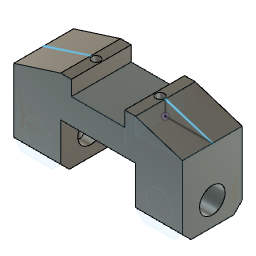
Antena (Autodesk Fusion 360 design; units mm, degrees)
Autodesk Fusion 360 part; units mm, degrees
sketch "Sketch1" plane through (0, 0, 0) normal (0, 0, 1) x (1, 0, 0)
  line L0 (-125, 140) -> (125, 140)
  line L1 (125, 140) -> (125, -140)
  line L2 (125, -140) -> (-125, -140)
  line L3 (-125, -140) -> (-125, 140)
  line L4 (-125, 140) -> (-175, 140)
  line L5 (-175, 140) -> (-175, -140)
  line L6 (-175, -140) -> (-125, -140)
  line L7 (-125, -140) -> (-125, 140)
  line L8 (-175, 140) -> (-425, 140)
  line L9 (-425, 140) -> (-425, -140)
  line L10 (-425, -140) -> (-175, -140)
  line L11 (-175, -140) -> (-175, 140)
  line L12 (125, 140) -> (175, 140)
  line L13 (175, 140) -> (175, -140)
  line L14 (175, -140) -> (125, -140)
  line L15 (125, -140) -> (125, 140)
  line L16 (175, 140) -> (425, 140)
  line L17 (425, 140) -> (425, -140)
  line L18 (425, -140) -> (175, -140)
  line L19 (175, -140) -> (175, 140)
  point P0 (-125, 140)
  dimension "d1" = 250
  dimension "d2" = 280
  dimension "d3" = 50
  dimension "d4" = 280
  dimension "d5" = 250
  dimension "d6" = 280
  dimension "d7" = 50
  dimension "d8" = 280
  dimension "d9" = 250
  dimension "d10" = 280
  constraint horizontal L0
  constraint vertical L1
  constraint horizontal L2
  constraint vertical L3
  constraint coincident P0 L0.start
  constraint horizontal L4
  constraint vertical L5
  constraint horizontal L6
  constraint vertical L7
  constraint horizontal L8
  constraint vertical L9
  constraint horizontal L10
  constraint vertical L11
  constraint horizontal L12
  constraint vertical L13
  constraint horizontal L14
  constraint vertical L15
  constraint horizontal L16
  constraint vertical L17
  constraint horizontal L18
  constraint vertical L19
  measures "d1" distance of P0 L0.end
  measures "d2" distance of P0 L2.end
  measures "d3" distance of P0 L4.end
  measures "d4" distance of P0 L2.end
  measures "d5" distance of L4.end L8.end
  measures "d6" distance of L4.end L5.end
  measures "d7" distance of L0.end L12.end
  measures "d8" distance of L0.end L1.end
  measures "d9" distance of L12.end L16.end
  measures "d10" distance of L12.end L13.end
extrude "Extrude1" add sketch "Sketch1" against normal blind 60 contours L0 L1 L2 L3 L7 L15 makes body 1
sketch "Sketch2" plane through (125, 0, 0) normal (1, 0, 0) x (0, 1, 0)
  line L0 (140, 0) -> (-140, 0)
  line L1 (-140, 0) -> (-140, -60)
  line L2 (-140, -60) -> (140, -60)
  line L3 (140, -60) -> (140, 0)
sketch "Sketch3" plane through (0, 0, 0) normal (0, 0, 1) x (1, 0, 0)
  line L0 (-125, 140) -> (-175, 140)
  line L1 (-175, 140) -> (-175, -140)
  line L2 (-175, -140) -> (-125, -140)
  line L3 (-125, -140) -> (-125, 140)
  line L4 (125, 140) -> (175, 140)
  line L5 (175, 140) -> (175, -140)
  line L6 (175, -140) -> (125, -140)
  line L7 (125, -140) -> (125, 140)
  dimension "d13" = 50
  dimension "d14" = 280
  dimension "d15" = 50
  dimension "d16" = 280
  constraint horizontal L0
  constraint vertical L1
  constraint horizontal L2
  constraint vertical L3
  constraint horizontal L4
  constraint vertical L5
  constraint horizontal L6
  constraint vertical L7
  measures "d13" distance of L0.start L0.end
  measures "d14" distance of L0.start L2.end
  measures "d15" distance of L4.start L4.end
  measures "d16" distance of L4.start L6.end
extrude "Extrude2" add sketch "Sketch3" along normal blind 70 separate body makes body 2 at (-125, -46.6667, 23.3333) makes body 3 at (175, 46.6667, 23.3333)
extrude "Extrude3" add 1 faces at (141.6667, 46.6667, 0) along direction (0, 0, -1) blind 60 on bodies 3 bodies 3 2 1
extrude "Extrude4" add 1 faces at (-158.3333, 46.6667, 0) along direction (0, 0, -1) blind 60 on bodies 2 bodies 2 3
sketch "Sketch4" plane through (0, 0, 0) normal (0, 0, 1) x (1, 0, 0)
  line L0 (-175, 140) -> (-395, 140)
  line L1 (-395, 140) -> (-395, -140)
  line L2 (-395, -140) -> (-175, -140)
  line L3 (-175, -140) -> (-175, 140)
  line L4 (175, 140) -> (395, 140)
  line L5 (395, 140) -> (395, -140)
  line L6 (395, -140) -> (175, -140)
  line L7 (175, -140) -> (175, 140)
  dimension "d23" = 220
  dimension "d24" = 280
  dimension "d25" = 220
  dimension "d26" = 280
  constraint horizontal L0
  constraint vertical L1
  constraint horizontal L2
  constraint vertical L3
  constraint horizontal L4
  constraint vertical L5
  constraint horizontal L6
  constraint vertical L7
  measures "d23" distance of L0.start L0.end
  measures "d24" distance of L0.start L2.end
  measures "d25" distance of L4.start L4.end
  measures "d26" distance of L4.start L6.end
extrude "Extrude5" add sketch "Sketch4" against normal blind 60 bodies 2
sketch "Sketch5" plane through (0, 0, 0) normal (0, 1, 0) x (1, 0, 0)
  line L0 (-175, -70) -> (-395, 0)
  line L1 (395, 0) -> (175, -70)
  line L2 (175, -70) -> (395, 0)
  line L3 (-175, -70) -> (-395, 0)
  constraint parallel L1 L2
sketch "Sketch6" plane through (0, 0, 0) normal (0, 0, 1) x (-1, 0, 0)
  line L0 (-175, 140) -> (-395, 140)
  line L1 (-395, 140) -> (-395, -140)
  line L2 (-395, -140) -> (-175, -140)
  line L3 (-175, -140) -> (-175, 140)
  line L4 (-175, 0) -> (-395, 0)
  constraint midpoint L3 L4.start
  constraint midpoint L1 L4.end
sketch "Sketch7" plane through (175, 0, 0) normal (1, 0, 0) x (0, 1, 0)
  line L0 (-140, 0) -> (140, 0)
  line L1 (140, 0) -> (140, 70)
  line L2 (140, 70) -> (-140, 70)
  line L3 (-140, 70) -> (-140, 0)
  line L4 (0, 70) -> (0, 0)
  constraint midpoint L2 L4.start
  constraint coincident L4.end origin
sketch "Sketch8" plane through (0, 0, 0) normal (0, 1, 0) x (1, 0, 0)
sketch "Sketch9" plane through (0, 0, 0) normal (0, 0, 1) x (-1, 0, 0)
sketch "Sketch10" plane through (0, -140, 0) normal (0, -1, 0) x (1, 0, 0)
  line L0 (-125, 0) -> (-125, 70)
  line L1 (-125, 70) -> (-175, 70)
  line L2 (-175, 70) -> (-175, 0)
  line L3 (-175, 0) -> (-395, 0)
  line L4 (-395, 0) -> (-395, -60)
  line L5 (-395, -60) -> (395, -60)
  line L6 (395, -60) -> (395, 0)
  line L7 (395, 0) -> (175, 0)
  line L8 (175, 0) -> (175, 70)
  line L9 (175, 70) -> (125, 70)
  line L10 (125, 70) -> (125, 0)
  line L11 (125, 0) -> (-125, 0)
  line L12 (175, 70) -> (395, 0)
  constraint coincident L8.end L9.start
  constraint coincident L6.end L7.start
extrude "Extrude6" add sketch "Sketch10" against normal blind 280 contours L7 L8 L12 bodies 2
sketch "Sketch11" plane through (0, -140, 0) normal (0, -1, 0) x (1, 0, 0)
  line L0 (-125, 0) -> (-125, 70)
  line L1 (-125, 70) -> (-175, 70)
  line L2 (-175, 70) -> (-175, 0)
  line L3 (-175, 0) -> (-395, 0)
  line L4 (-395, 0) -> (-395, -60)
  line L5 (-395, -60) -> (395, -60)
  line L6 (395, -60) -> (395, 0)
  line L7 (395, 0) -> (175, 70)
  line L8 (175, 70) -> (125, 70)
  line L9 (125, 70) -> (125, 0)
  line L10 (125, 0) -> (-125, 0)
  line L11 (-175, 70) -> (-395, 0)
  constraint coincident L1.end L2.start
  constraint coincident L3.end L4.start
extrude "Extrude7" add sketch "Sketch11" against normal blind 280 contours L2 L3 L11 bodies 2
sketch "Sketch12" plane through (0, 0, 0) normal (0, 0, 1) x (-1, 0, 0)
  line L0 (125, 140) -> (-125, 140)
  line L1 (-125, 140) -> (-125, -140)
  line L2 (-125, -140) -> (125, -140)
  line L3 (125, -140) -> (125, 140)
sketch "Sketch13" plane through (0, 0, -60) normal (0, 0, -1) x (1, 0, 0)
  line L0 (395, 140) -> (-395, 140)
  line L1 (-395, 140) -> (-395, -140)
  line L2 (-395, -140) -> (395, -140)
  line L3 (395, -140) -> (395, 140)
  line L4 (-395, 140) -> (-175, 140)
  line L5 (-175, 140) -> (-175, -140)
  line L6 (-175, -140) -> (-395, -140)
  line L7 (-395, -140) -> (-395, 140)
  line L8 (395, 140) -> (175, 140)
  line L9 (175, 140) -> (175, -140)
  line L10 (175, -140) -> (395, -140)
  line L11 (395, -140) -> (395, 140)
  dimension "d33" = 220
  dimension "d34" = 280
  dimension "d35" = 220
  dimension "d36" = 280
  constraint horizontal L4
  constraint vertical L5
  constraint horizontal L6
  constraint vertical L7
  constraint coincident L0.end L1.start
  constraint horizontal L8
  constraint vertical L9
  constraint horizontal L10
  constraint vertical L11
  constraint coincident L0.start L3.end
  measures "d33" distance of L0.end L4.end
  measures "d34" distance of L0.end L1.end
  measures "d35" distance of L0.start L8.end
  measures "d36" distance of L0.start L2.end
extrude "Extrude8" add sketch "Sketch13" along normal blind 240 contours L0 L2 L3 L8 L9 L10 L11 | L0 L1 L2 L4 L5 L6 L7 bodies 2
extrude "Extrude9" add 1 faces at (-58.3333, 46.6667, -60) along direction (0, 0, -1) blind 40 on bodies 2 bodies 2
extrude "Extrude10" add 1 faces at (-58.3333, 46.6667, -100) along direction (0, 0, -1) blind 20 on bodies 2 bodies 2
form "Form1" [no effect]
sketch "Sketch14" plane through (0, 0, -300) normal (0, 0, -1) x (1, 0, 0)
  line L0 (-395, -140) -> (-175, -140)
  line L1 (-175, -140) -> (-175, 140)
  line L2 (-175, 140) -> (-395, 140)
  line L3 (-395, 140) -> (-395, -140)
  line L4 (-395, 140) -> (-355, 140)
  line L5 (-355, 140) -> (-355, -140)
  line L6 (-355, -140) -> (-395, -140)
  line L7 (-395, -140) -> (-395, 140)
  line L8 (-175, 140) -> (-215, 140)
  line L9 (-215, 140) -> (-215, -140)
  line L10 (-215, -140) -> (-175, -140)
  line L11 (-175, -140) -> (-175, 140)
  line L12 (395, 140) -> (355, 140)
  line L13 (355, 140) -> (355, -140)
  line L14 (355, -140) -> (395, -140)
  line L15 (395, -140) -> (395, 140)
  line L16 (175, 140) -> (215, 140)
  line L17 (215, 140) -> (215, -140)
  line L18 (215, -140) -> (175, -140)
  line L19 (175, -140) -> (175, 140)
  dimension "d43" = 40
  dimension "d44" = 280
  dimension "d45" = 40
  dimension "d46" = 280
  dimension "d47" = 40
  dimension "d48" = 280
  dimension "d49" = 40
  dimension "d50" = 280
  constraint horizontal L4
  constraint vertical L5
  constraint horizontal L6
  constraint vertical L7
  constraint coincident L2.end L3.start
  constraint horizontal L8
  constraint vertical L9
  constraint horizontal L10
  constraint vertical L11
  constraint coincident L1.end L2.start
  constraint horizontal L12
  constraint vertical L13
  constraint horizontal L14
  constraint vertical L15
  constraint horizontal L16
  constraint vertical L17
  constraint horizontal L18
  constraint vertical L19
  measures "d43" distance of L2.end L4.end
  measures "d44" distance of L2.end L0.start
  measures "d45" distance of L1.end L8.end
  measures "d46" distance of L1.end L0.end
  measures "d47" distance of L12.start L12.end
  measures "d48" distance of L12.start L14.end
  measures "d49" distance of L16.start L16.end
  measures "d50" distance of L16.start L18.end
sketch "Sketch15" plane through (0, 0, -300) normal (0, 0, -1) x (1, 0, 0)
  line L0 (395, -140) -> (395, 140)
  line L1 (395, 140) -> (175, 140)
  line L2 (175, 140) -> (175, -140)
  line L3 (175, -140) -> (395, -140)
  line L4 (175, -140) -> (215, -140)
  line L5 (215, -140) -> (215, 140)
  line L6 (215, 140) -> (175, 140)
  line L7 (175, 140) -> (175, -140)
  line L8 (395, -140) -> (355, -140)
  line L9 (355, -140) -> (355, 140)
  line L10 (355, 140) -> (395, 140)
  line L11 (395, 140) -> (395, -140)
  dimension "d51" = 40
  dimension "d52" = 280
  dimension "d53" = 40
  dimension "d54" = 280
  constraint horizontal L4
  constraint vertical L5
  constraint horizontal L6
  constraint vertical L7
  constraint coincident L2.end L3.start
  constraint horizontal L8
  constraint vertical L9
  constraint horizontal L10
  constraint vertical L11
  constraint coincident L0.start L3.end
  measures "d51" distance of L2.end L4.end
  measures "d52" distance of L2.end L1.end
  measures "d53" distance of L0.start L8.end
  measures "d54" distance of L0.start L0.end
extrude "Extrude11" add sketch "Sketch14" sketch "Sketch15" along normal blind 40 contours L0 L2 L5 L9 of sketch 2 contours L1 L3 L5 L9 bodies 2
sketch "Sketch16" plane through (0, -140, 0) normal (0, -1, 0) x (1, 0, 0)
  line L0 (-125, 0) -> (-125, 70)
  line L1 (-125, 70) -> (-175, 70)
  line L2 (-175, 70) -> (-395, 0)
  line L3 (-395, 0) -> (-395, -300)
  line L4 (-395, -300) -> (-355, -300)
  line L5 (-355, -300) -> (-355, -340)
  line L6 (-355, -340) -> (-215, -340)
  line L7 (-215, -340) -> (-215, -300)
  line L8 (-215, -300) -> (-175, -300)
  line L9 (-175, -300) -> (-175, -120)
  line L10 (-175, -120) -> (175, -120)
  line L11 (175, -120) -> (175, -300)
  line L12 (175, -300) -> (215, -300)
  line L13 (215, -300) -> (215, -340)
  line L14 (215, -340) -> (355, -340)
  line L15 (355, -340) -> (355, -300)
  line L16 (355, -300) -> (395, -300)
  line L17 (395, -300) -> (395, 0)
  line L18 (395, 0) -> (175, 70)
  line L19 (175, 70) -> (125, 70)
  line L20 (125, 70) -> (125, 0)
  line L21 (125, 0) -> (-125, 0)
  line L22 (-355, -340) -> (-395, -300)
  line L23 (-215, -340) -> (-175, -300)
  line L24 (215, -340) -> (175, -300)
  line L25 (355, -340) -> (395, -300)
  constraint coincident L5.end L6.start
  constraint coincident L3.end L4.start
  constraint coincident L6.end L7.start
  constraint coincident L8.end L9.start
  constraint coincident L13.end L14.start
  constraint coincident L11.end L12.start
  constraint coincident L14.end L15.start
  constraint coincident L16.end L17.start
extrude "Extrude12" add sketch "Sketch16" against normal blind 280 contours L4 L5 L22 | L15 L16 L25 | L7 L8 L23 | L12 L13 L24 bodies 2
sketch "Sketch17" plane through (0, -140, 0) normal (0, -1, 0) x (1, 0, 0)
  line L0 (-125, 0) -> (-125, 70)
  line L1 (-125, 70) -> (-175, 70)
  line L2 (-175, 70) -> (-395, 0)
  line L3 (-395, 0) -> (-395, -300)
  line L4 (-395, -300) -> (-355, -340)
  line L5 (-355, -340) -> (-215, -340)
  line L6 (-215, -340) -> (-175, -300)
  line L7 (-175, -300) -> (-175, -120)
  line L8 (-175, -120) -> (175, -120)
  line L9 (175, -120) -> (175, -300)
  line L10 (175, -300) -> (215, -340)
  line L11 (215, -340) -> (355, -340)
  line L12 (355, -340) -> (395, -300)
  line L13 (395, -300) -> (395, 0)
  line L14 (395, 0) -> (175, 70)
  line L15 (175, 70) -> (125, 70)
  line L16 (125, 70) -> (125, 0)
  line L17 (125, 0) -> (-125, 0)
  line L18 (-285, -340) -> (-285, -230)
  circle A0 centre (-285, -230) radius 60
  line L19 (285, -340) -> (285, -230)
  circle A1 centre (285, -230) radius 60
  point P0 (-285, -340)
  point P1 (285, -340)
  dimension "d59" = 110
  dimension "d60" = 120
  dimension "d61" = 110
  dimension "d62" = 120
  constraint midpoint L5 P0
  constraint vertical L18
  constraint coincident P0 L18.start
  constraint coincident L18.end A0.centre
  constraint midpoint L11 P1
  constraint vertical L19
  constraint coincident P1 L19.start
  constraint coincident L19.end A1.centre
  measures "d59" distance of P0 L18.end
  measures "d60" diameter of A0
  measures "d61" distance of P1 L19.end
  measures "d62" diameter of A1
extrude "Extrude13" cut sketch "Sketch17" against normal blind 280 contours A0 | A1 bodies 2
sketch "Sketch18" plane through (0, 0, 0) normal (0, 1, 0) x (1, 0, 0)
sketch "Sketch19" plane through (0, 0, 0) normal (0, 0, 1) x (1, 0, 0)
sketch "Sketch20" plane through (0, 0, 70) normal (0, 0, 1) x (-1, 0, 0)
  line L0 (-125, 140) -> (-175, 140)
  line L1 (-175, 140) -> (-175, -140)
  line L2 (-175, -140) -> (-125, -140)
  line L3 (-125, -140) -> (-125, 140)
  circle A0 centre (-150, 0) radius 20
  dimension "d65" = 40
  measures "d65" diameter of A0
sketch "Sketch21" plane through (0, 0, 70) normal (0, 0, 1) x (-1, 0, 0)
  line L0 (125, 140) -> (125, -140)
  line L1 (125, -140) -> (175, -140)
  line L2 (175, -140) -> (175, 140)
  line L3 (175, 140) -> (125, 140)
  circle A0 centre (150, 0) radius 20
  dimension "d66" = 40
  measures "d66" diameter of A0
extrude "Extrude14" cut sketch "Sketch20" sketch "Sketch21" against normal blind 190 contours A0 of sketch 2 contours A0 bodies 2
sketch "Sketch22" plane through (0, -140, 0) normal (0, -1, 0) x (1, 0, 0)
  circle A0 centre (-285, -230) radius 60
  circle A1 centre (285, -230) radius 60
  line L0 (-125, 0) -> (-125, 70)
  line L1 (-125, 70) -> (-175, 70)
  line L2 (-175, 70) -> (-395, 0)
  line L3 (-395, 0) -> (-395, -300)
  line L4 (-395, -300) -> (-355, -340)
  line L5 (-355, -340) -> (-215, -340)
  line L6 (-215, -340) -> (-175, -300)
  line L7 (-175, -300) -> (-175, -120)
  line L8 (-175, -120) -> (175, -120)
  line L9 (175, -120) -> (175, -300)
  line L10 (175, -300) -> (215, -340)
  line L11 (215, -340) -> (355, -340)
  line L12 (355, -340) -> (395, -300)
  line L13 (395, -300) -> (395, 0)
  line L14 (395, 0) -> (175, 70)
  line L15 (175, 70) -> (125, 70)
  line L16 (125, 70) -> (125, 0)
  line L17 (125, 0) -> (-125, 0)
delete_face "DeleteFace1" 1 faces at (225.2982, 46.6667, -224.0259) on bodies 2
delete_face "DeleteFace2" 1 faces at (-344.7018, 46.6667, -224.0259) on bodies 2
sketch "Sketch23" plane through (0, 0, -340) normal (0, 0, -1) x (1, 0, 0)
  line L0 (-355, 140) -> (-355, -140)
  line L1 (-355, -140) -> (-215, -140)
  line L2 (-215, -140) -> (-215, 140)
  line L3 (-215, 140) -> (-355, 140)
  line L4 (-355, -140) -> (-395, -140)
  line L5 (-395, -140) -> (-395, 140)
  line L6 (-395, 140) -> (-355, 140)
  line L7 (-355, 140) -> (-355, -140)
  line L8 (-215, -140) -> (-175, -140)
  line L9 (-175, -140) -> (-175, 140)
  line L10 (-175, 140) -> (-215, 140)
  line L11 (-215, 140) -> (-215, -140)
  dimension "d69" = 40
  dimension "d70" = 280
  dimension "d71" = 40
  dimension "d72" = 280
  constraint horizontal L4
  constraint vertical L5
  constraint horizontal L6
  constraint vertical L7
  constraint coincident L0.end L1.start
  constraint horizontal L8
  constraint vertical L9
  constraint horizontal L10
  constraint vertical L11
  constraint coincident L1.end L2.start
  measures "d69" distance of L0.end L4.end
  measures "d70" distance of L0.end L0.start
  measures "d71" distance of L1.end L8.end
  measures "d72" distance of L1.end L2.end
extrude "Extrude15" cut sketch "Sketch23" against normal blind 40 bodies 2
sketch "Sketch24" plane through (0, 0, -340) normal (0, 0, -1) x (1, 0, 0)
  line L0 (215, -140) -> (355, -140)
  line L1 (355, -140) -> (355, 140)
  line L2 (355, 140) -> (215, 140)
  line L3 (215, 140) -> (215, -140)
  line L4 (355, -140) -> (395, -140)
  line L5 (395, -140) -> (395, 140)
  line L6 (395, 140) -> (355, 140)
  line L7 (355, 140) -> (355, -140)
  line L8 (215, 140) -> (175, 140)
  line L9 (175, 140) -> (175, -140)
  line L10 (175, -140) -> (215, -140)
  line L11 (215, -140) -> (215, 140)
  dimension "d75" = 40
  dimension "d76" = 40
  dimension "d77" = 280
  constraint horizontal L4
  constraint vertical L5
  constraint horizontal L6
  constraint vertical L7
  constraint coincident L0.end L1.start
  constraint horizontal L8
  constraint vertical L9
  constraint horizontal L10
  constraint vertical L11
  constraint coincident L2.end L3.start
  measures "d75" distance of L0.end L4.end
  measures "d76" distance of L2.end L8.end
  measures "d77" distance of L2.end L0.start
extrude "Extrude16" cut sketch "Sketch24" against normal blind 40 bodies 2
sketch "Sketch25" plane through (0, 0, -300) normal (0, 0, -1) x (1, 0, 0)
  line L0 (175, -140) -> (395, -140)
  line L1 (395, -140) -> (395, 140)
  line L2 (395, 140) -> (175, 140)
  line L3 (175, 140) -> (175, -140)
  line L4 (175, -140) -> (395, -140)
  line L5 (395, -140) -> (395, -100)
  line L6 (395, -100) -> (175, -100)
  line L7 (175, -100) -> (175, -140)
  line L8 (175, 140) -> (395, 140)
  line L9 (395, 140) -> (395, 100)
  line L10 (395, 100) -> (175, 100)
  line L11 (175, 100) -> (175, 140)
  dimension "d80" = 220
  dimension "d81" = 40
  dimension "d82" = 220
  dimension "d83" = 40
  constraint horizontal L4
  constraint vertical L5
  constraint horizontal L6
  constraint vertical L7
  constraint coincident L0.start L3.end
  constraint horizontal L8
  constraint vertical L9
  constraint horizontal L10
  constraint vertical L11
  constraint coincident L2.end L3.start
  measures "d80" distance of L0.start L0.end
  measures "d81" distance of L0.start L6.end
  measures "d82" distance of L2.end L1.end
  measures "d83" distance of L2.end L10.end
extrude "Extrude17" add sketch "Sketch25" along normal blind 40 contours L1 L3 L6 L10 bodies 2
sketch "Sketch26" plane through (0, 0, -300) normal (0, 0, -1) x (1, 0, 0)
  line L0 (-395, -140) -> (-175, -140)
  line L1 (-175, -140) -> (-175, 140)
  line L2 (-175, 140) -> (-395, 140)
  line L3 (-395, 140) -> (-395, -140)
  line L4 (-395, -140) -> (-175, -140)
  line L5 (-175, -140) -> (-175, -100)
  line L6 (-175, -100) -> (-395, -100)
  line L7 (-395, -100) -> (-395, -140)
  line L8 (-395, 140) -> (-175, 140)
  line L9 (-175, 140) -> (-175, 100)
  line L10 (-175, 100) -> (-395, 100)
  line L11 (-395, 100) -> (-395, 140)
  dimension "d86" = 220
  dimension "d87" = 40
  dimension "d88" = 220
  dimension "d89" = 40
  constraint horizontal L4
  constraint vertical L5
  constraint horizontal L6
  constraint vertical L7
  constraint coincident L0.start L3.end
  constraint horizontal L8
  constraint vertical L9
  constraint horizontal L10
  constraint vertical L11
  constraint coincident L2.end L3.start
  measures "d86" distance of L0.start L0.end
  measures "d87" distance of L0.start L6.end
  measures "d88" distance of L2.end L1.end
  measures "d89" distance of L2.end L10.end
extrude "Extrude18" add sketch "Sketch26" along normal blind 40 contours L1 L3 L6 L10 bodies 2
sketch "Sketch27" plane through (-175, 0, 0) normal (1, 0, 0) x (0, 1, 0)
  line L0 (140, -120) -> (-140, -120)
  line L1 (-140, -120) -> (-140, -300)
  line L2 (-140, -300) -> (-100, -300)
  line L3 (-100, -300) -> (-100, -340)
  line L4 (-100, -340) -> (100, -340)
  line L5 (100, -340) -> (100, -300)
  line L6 (100, -300) -> (140, -300)
  line L7 (140, -300) -> (140, -120)
  line L8 (-100, -340) -> (-140, -300)
  line L9 (100, -340) -> (140, -300)
  constraint coincident L3.end L4.start
  constraint coincident L1.end L2.start
  constraint coincident L4.end L5.start
  constraint coincident L6.end L7.start
sketch "Sketch28" plane through (395, 0, 0) normal (1, 0, 0) x (0, 1, 0)
  line L0 (140, 0) -> (-140, 0)
  line L1 (-140, 0) -> (-140, -300)
  line L2 (-140, -300) -> (-100, -300)
  line L3 (-100, -300) -> (-100, -340)
  line L4 (-100, -340) -> (100, -340)
  line L5 (100, -340) -> (100, -300)
  line L6 (100, -300) -> (140, -300)
  line L7 (140, -300) -> (140, 0)
  line L8 (-100, -340) -> (-140, -300)
  line L9 (100, -340) -> (140, -300)
  constraint coincident L3.end L4.start
  constraint coincident L1.end L2.start
  constraint coincident L4.end L5.start
  constraint coincident L6.end L7.start
extrude "Extrude19" add sketch "Sketch28" against normal blind 220 contours L5 L6 L9 | L2 L3 L8 bodies 2
extrude "Extrude20" add sketch "Sketch27" against normal blind 220 contours L5 L6 L9 | L2 L3 L8 bodies 2
sketch "Sketch29" plane through (-395, 0, 0) normal (-1, 0, 0) x (0, -1, 0)
  line L0 (140, 0) -> (-140, 0)
  line L1 (-140, 0) -> (-140, -300)
  line L2 (-140, -300) -> (-100, -340)
  line L3 (-100, -340) -> (100, -340)
  line L4 (100, -340) -> (140, -300)
  line L5 (140, -300) -> (140, 0)
  line L6 (0, -340) -> (0, -230)
  circle A0 centre (0, -230) radius 60
  dimension "d96" = 110
  dimension "d97" = 120
  constraint midpoint L3 L6.start
  constraint perpendicular L3 L6
  constraint coincident L6.end A0.centre
  measures "d96" distance of L6.start L6.end
  measures "d97" diameter of A0
sketch "Sketch30" plane through (395, 0, 0) normal (1, 0, 0) x (0, 1, 0)
  line L0 (140, 0) -> (-140, 0)
  line L1 (-140, 0) -> (-140, -300)
  line L2 (-140, -300) -> (-100, -340)
  line L3 (-100, -340) -> (100, -340)
  line L4 (100, -340) -> (140, -300)
  line L5 (140, -300) -> (140, 0)
sketch "Sketch31" plane through (395, 0, -170) normal (1, 0, 0) x (0, 1, 0)
  line L0 (0, -170) -> (0, -60)
  circle A0 centre (0, -60) radius 60
  dimension "d98" = 120
  constraint vertical L0
  constraint coincident L0.end A0.centre
  measures "d98" diameter of A0
extrude "Extrude21" cut sketch "Sketch31" against normal blind 220 bodies 2
extrude "Extrude22" cut sketch "Sketch29" against normal blind 220 contours A0 bodies 2
sketch "Sketch32" plane through (0, 0, -340) normal (0, 0, -1) x (1, 0, 0)
  line L0 (395, -100) -> (395, 100)
  line L1 (395, 100) -> (175, 100)
  line L2 (175, 100) -> (175, -100)
  line L3 (175, -100) -> (395, -100)
  line L4 (175, 0) -> (265, 0)
  circle A0 centre (265, 0) radius 40
  line L5 (-175, 0) -> (-265, 0)
  circle A1 centre (-265, 0) radius 40
  dimension "d108" = 90
  dimension "d109" = 80
  dimension "d110" = 90
  dimension "d111" = 80
  constraint midpoint L2 L4.start
  constraint perpendicular L2 L4
  constraint coincident L4.end A0.centre
  constraint horizontal L5
  constraint coincident L5.end A1.centre
  measures "d108" distance of L4.start L4.end
  measures "d109" diameter of A0
  measures "d110" distance of L5.start L5.end
  measures "d111" diameter of A1
extrude "Extrude23" cut sketch "Sketch32" against normal blind 100 contours A0 | A1 bodies 2
